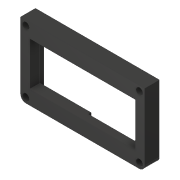
# Autodesk Inventor part: Faceplate
Saved by Autodesk Inventor 2020 (Build 240168000, 168)
## iProperties
Created: 2018-09-01
Part Number: Faceplate
Material: Acetal Resin, Black
Document SubType Name: Modeling
Designer: amsmi
Density: 1.425 g/cm^3
Appearance: Smooth - Black
Mass: 55.3777 g
Surface Area: 172.295 cm^2
Volume: 38.8616 cm^3
Author: amsmi
Autodesk Inventor part; units mm, degrees
ref_plane "YZ Plane" through (0, 0, 0) normal (1, 0, 0) x (0, 1, 0)
ref_plane "XZ Plane" through (0, 0, 0) normal (0, 1, 0) x (-1, 0, 0)
ref_plane "XY Plane" through (0, 0, 0) normal (0, 0, 1) x (1, 0, 0)
sketch "Sketch1" plane through (0, 0, 0) normal (0, 0, 1) x (1, 0, 0)
  line L0 (48.7934, -20.1549) -> (-48.7934, -20.1549)
  line L1 (-48.7934, -20.1549) -> (-48.7934, 20.1549)
  line L2 (-48.7934, 20.1549) -> (48.7934, 20.1549)
  line L3 (48.7934, 20.1549) -> (48.7934, -20.1549)
  line L4 (-57.15, -33.2867) -> (57.15, -33.2867)
  line L5 (57.15, -33.2867) -> (57.15, 33.2867)
  line L6 (57.15, 33.2867) -> (-57.15, 33.2867)
  line L7 (-57.15, 33.2867) -> (-57.15, -33.2867)
  line L8 (-57.15, -33.2867) -> (57.15, 33.2867) construction
  line L9 (57.15, -33.2867) -> (-57.15, 33.2867) construction
  point P0 (0, 0)
  point P1 (0, 20.1549)
  point P2 (0, 0)
  point P3 (0, 0)
  point P4 (-48.7934, 0)
  dimension "d38" = 40.3098
  dimension "d39" = 97.5868
  constraints: 20 end point, 6 midpoint, 3 horizontal, 2 parallel, 2 vertical, 1 horizontal alignment, 1 perpendicular, 1 vertical alignment
  measures "d38" distance of L0.end L1.end
  measures "d39" distance of L0.start L0.end
extrude "Extrusion1" add sketch "Sketch1" against normal blind 9.4488
ref_plane "Work Plane14" through (57.15, 33.2867, -9.4488) normal (0, 0, -1) x (-1, 0, 0)
sketch "Sketch2" plane through (57.15, 33.2867, -9.4488) normal (0, 0, -1) x (-1, 0, 0)
  line L0 (16.1036, -63.3984) -> (58.8264, -63.3984)
  line L1 (58.8264, -63.3984) -> (58.8264, -53.4416)
  line L2 (58.8264, -53.4416) -> (16.1036, -53.4416)
  line L3 (16.1036, -53.4416) -> (16.1036, -63.3984)
  line L4 (8.3566, -53.4416) -> (8.3566, -13.1318) projected
  dimension "d35" = 42.7228
  dimension "d36" = 9.9568
  dimension "d40" = 7.747
  constraints: 8 end point, 2 parallel, 1 horizontal, 1 horizontal alignment, 1 perpendicular
  measures "d35" distance between parallel lines of L3 L1
  measures "d36" distance of L2.end L0.start
  measures "d40" distance between parallel lines of L4 L3
extrude "Extrusion2" cut sketch "Sketch2" against normal blind 2.54
ref_plane "Work Plane15" through (57.15, 33.2867, -9.4488) normal (0, 0, -1) x (-1, 0, 0)
sketch "Sketch8" plane through (0, 0, -9.4488) normal (0, 0, -1) x (-1, 0, 0)
  line L0 (57.15, 33.2867) -> (-57.15, 33.2867) projected
  line L1 (-57.15, 33.2867) -> (-57.15, -33.2867) projected
  line L2 (-57.15, -33.2867) -> (57.15, -33.2867) projected
  line L3 (57.15, -33.2867) -> (57.15, 33.2867) projected
  line L4 (-49.5554, 30.6197) -> (49.5554, 30.6197)
  line L5 (49.5554, 30.6197) -> (49.5554, -30.6197)
  line L6 (49.5554, -30.6197) -> (-49.5554, -30.6197)
  line L7 (-49.5554, -30.6197) -> (-49.5554, 30.6197)
  point P0 (0, 0)
  dimension "d53" = 7.5946
  dimension "d54" = 61.2394
  dimension "d55" = 2.667
  dimension "d56" = 99.1108
  constraints: 8 end point, 2 parallel, 1 horizontal, 1 perpendicular
  measures "d53" distance between parallel lines of L1 L7
  measures "d54" distance of L6.end L4.start
  measures "d55" distance between parallel lines of L2 L6
  measures "d56" distance of L5.end L6.end
extrude "Extrusion6" add sketch "Sketch8" along normal blind 4.2164
sketch "Sketch4" plane through (0, 0, 0) normal (0, 0, 1) x (1, 0, 0)
  line L0 (57.15, -33.2867) -> (-57.15, -33.2867) construction
  line L1 (57.15, 33.2867) -> (57.15, -33.2867) construction
  line L2 (-57.15, 33.2867) -> (57.15, 33.2867) construction
  line L3 (-57.15, -33.2867) -> (-57.15, 33.2867) construction
  line L4 (-52.3875, -28.5242) -> (52.3875, -28.5242) construction
  line L5 (52.3875, -28.5242) -> (52.3875, 28.5242) construction
  line L6 (52.3875, 28.5242) -> (-52.3875, 28.5242) construction
  line L7 (-52.3875, 28.5242) -> (-52.3875, -28.5242) construction
  point P0 (0, 0)
  dimension "d11" = 4.7625
  constraints: 8 end point, 4 coincident, 3 other
  measures "d11" distance between parallel lines of L0 L4
hole "Hole1" at (52.3875, -28.5242, 0) at (52.3875, 28.5242, 0) at (-52.3875, 28.5242, 0) at (-52.3875, -28.5242, 0) direction (0, 0, -1) diameter 3.048 end through all counterbore diameter 6.35 counterbore depth 0.0254
sketch "Sketch5" plane through (52.3875, -28.5242, -0.0254) normal (0, 0, 1) x (1, 0, 0)
  circle A0 centre (0, 0) radius 3.175 projected
  circle A1 centre (0, 0) radius 1.524 projected
  circle A2 centre (0, 57.0484) radius 3.175 projected
  circle A3 centre (0, 57.0484) radius 1.524 projected
  circle A4 centre (-104.775, 57.0484) radius 3.175 projected
  circle A5 centre (-104.775, 57.0484) radius 1.524 projected
  circle A6 centre (-104.775, 0) radius 3.175 projected
  circle A7 centre (-104.775, 0) radius 1.524 projected
  point P0 (-52.3875, 28.5242)
extrude "Extrusion4" cut sketch "Sketch5" against normal up to surface (9.4234 mm away) contours A0 | A1 | A2 | A3 | A4 | A5 | A6 | A7
fillet "Fillet1" radius 4.7625 2 edges at (57.15, -33.2867, -6.8326) (-57.15, -33.2867, -6.8326)
ref_plane "Work Plane13" through (49.5554, 30.6197, -9.4488) normal (0, 0, -1) x (-1, 0, 0)
ref_plane "Work Plane5" through (0, 0, -1.5875) normal (0, 0, 1) x (1, 0, 0)
sketch "Sketch9" plane through (0, 0, -9.4488) normal (0, 0, -1) x (-1, 0, 0)
  line L0 (57.15, 33.2867) -> (-57.15, 33.2867) projected
  line L1 (-57.15, 33.2867) -> (-57.15, -28.5242) projected
  point P0 (0, 0)
  point P1 (-46.482, 27.5717)
  point P2 (-46.482, -27.4193)
  point P3 (46.482, 27.5717)
  point P4 (46.482, -27.4193)
  dimension "d60" = 5.715
  dimension "d61" = 10.668
  dimension "d62" = 92.964
  dimension "d63" = 54.991
  constraints: 2 horizontal alignment, 2 vertical alignment
  measures "d60" distance from line of L0 point (-46.482, 27.572)
  measures "d61" distance from line of L1 point (-46.482, 27.572)
  measures "d62" distance of point (46.482, 27.572) point (-46.482, 27.572)
  measures "d63" distance of point (-46.482, -27.419) point (-46.482, 27.572)
hole "Hole3" at (46.482, 27.5717, -9.4488) at (46.482, -27.4193, -9.4488) at (-46.482, 27.5717, -9.4488) at (-46.482, -27.4193, -9.4488) direction (0, 0, 1) diameter 2.2606 depth 6.35
equation "\"d23\" = 0.5 * Screw"
equation "\"Screw\" = 9.525"
body "Solid1"
